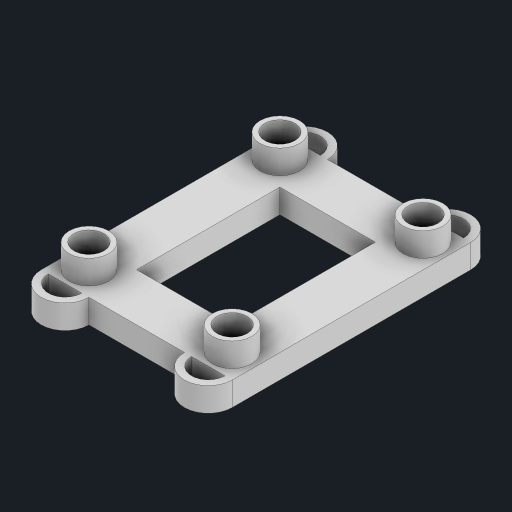
# Autodesk Inventor part: carriage_top
Saved by Autodesk Inventor 2024 (Build 280153000, 153)
## iProperties
Created: 2024-06-21
Part Number: carriage_top
Material: Generic
Document SubType Name: Modeling
Designer: mihir
Density: 1 g/cm^3
Appearance: Default
Author: mihir
Autodesk Inventor part; units mm, degrees
ref_plane "YZ Plane" through (0, 0, 0) normal (1, 0, 0) x (0, 1, 0)
ref_plane "XZ Plane" through (0, 0, 0) normal (0, 1, 0) x (-1, 0, 0)
ref_plane "XY Plane" through (0, 0, 0) normal (0, 0, 1) x (1, 0, 0)
sketch "Sketch1" plane through (0, 0, 0) normal (0, 1, 0) x (-1, 0, 0)
  line L0 (0, 0) -> (40, 0)
  line L1 (40, 0) -> (40, -50)
  line L2 (40, -50) -> (0, -50)
  line L3 (0, -50) -> (0, 0)
  line L4 (10, -10) -> (30, -10)
  line L5 (30, -10) -> (30, -40)
  line L6 (30, -40) -> (10, -40)
  line L7 (10, -40) -> (10, -10)
  line L8 (30, -25) -> (40, -25) construction
  line L9 (20, -10) -> (20, 0) construction
  arc A0 (40, 0) -> (30, 0) centre (35, 0) ccw
  arc A1 (10, 0) -> (0, 0) centre (5, 0) ccw
  arc A2 (38.5, 0) -> (31.5, 0) centre (35, 0) ccw
  arc A3 (8.5, 0) -> (1.5, 0) centre (5, 0) ccw
  arc A4 (30, -50) -> (40, -50) centre (35, -50) ccw
  arc A5 (0, -50) -> (10, -50) centre (5, -50) ccw
  arc A6 (31.5, -50) -> (38.5, -50) centre (35, -50) ccw
  arc A7 (1.5, -50) -> (8.5, -50) centre (5, -50) ccw
  dimension "d0" = 50
  dimension "d1" = 40
  dimension "d2" = 30
  dimension "d3" = 20
  dimension "d4" = 5
  dimension "d5" = 5
  dimension "d6" = 1.5
  dimension "d7" = 1.5
  constraints: 18 end point, 16 point on circle, 10 symmetric about line, 8 centre point, 4 coincident, 3 horizontal, 3 midpoint, 3 parallel, 2 tangent, 2 vertical, 1 perpendicular, 14 other
  measures "d0" distance of L2.end L3.end
  measures "d1" distance of L3.end L1.start
  measures "d2" distance of L6.end L4.start
  measures "d3" distance of L5.end L6.end
  measures "d4" radius of A0
  measures "d5" radius of A1
  measures "d6" radial gap between concentric circles of A0 A2
  measures "d7" radial gap between concentric circles of A1 A3
extrude "Extrusion1" add sketch "Sketch1" along normal blind 5 contours A1 L0 A3 | L0 L1 L2 L3 | L2 A7 A5 | A0 L0 A2 | L2 A6 A4
sketch "Sketch2" plane through (0, 5, 0) normal (0, 1, 0) x (1, 0, 0)
  line L0 (-30, 0) -> (-10, 0) construction
  line L1 (-10, 40) -> (-10, 10) construction
  line L2 (-10, 0) -> (-10, 10) construction
  line L3 (-10, 10) -> (0, 10) construction
  line L4 (-10, 10) -> (0, 0) construction
  arc A0 (-10, 0) -> (0, 0) centre (-5, 0) ccw construction
  line L5 (-10, 0) -> (0, 0) construction
  line L6 (-5, 0) -> (-5, 5) construction
  line L7 (-40, 50) -> (-40, 0) construction
  line L8 (-40, 25) -> (0, 25) construction
  line L9 (0, 0) -> (0, 50) construction
  line L10 (-20, 0) -> (-20, 50) construction
  line L11 (-10, 50) -> (-30, 50) construction
  circle A1 centre (-5, 5) radius 3.15
  circle A2 centre (-5, 5) radius 4.15
  circle A3 centre (-5, 45) radius 3.15
  circle A4 centre (-5, 45) radius 4.15
  circle A5 centre (-35, 5) radius 3.15
  circle A6 centre (-35, 5) radius 4.15
  circle A7 centre (-35, 45) radius 3.15
  circle A8 centre (-35, 45) radius 4.15
  dimension "d10" = 1
  dimension "d11" = 6.3
  constraints: 14 end point, 8 centre point, 6 symmetric about line, 5 coincident, 5 midpoint, 1 collinear, 1 horizontal, 1 perpendicular, 6 other
  measures "d10" radial gap between concentric circles of A2 A1
  measures "d11" diameter of A1
extrude "Extrusion2" add sketch "Sketch2" along normal blind 5
equation "\"d0\" = carriage_top_length"
equation "\"d1\" = carriage_top_width"
equation "\"d2\" = carriage_mount_cutout_length"
equation "\"d3\" = carriage_mount_cutout_width"
equation "\"d8\" = carriage_top_thickness"
equation "\"d10\" = carriage_mount_wall_thickness"
equation "\"d11\" = rod_diameter + rod_tolerance"
equation "\"d12\" = carriage_top_thickness"
equation "\"carriage_mount_cutout_length\" = 30"
equation "\"carriage_mount_cutout_width\" = 20"
equation "\"carriage_top_length\" = 50"
equation "\"carriage_top_width\" = 40"
equation "\"carriage_top_thickness\" = 5"
equation "\"carriage_mount_wall_thickness\" = 1"
equation "\"rod_diameter\" = 6"
equation "\"rod_tolerance\" = 0.3"
body "Solid1"
